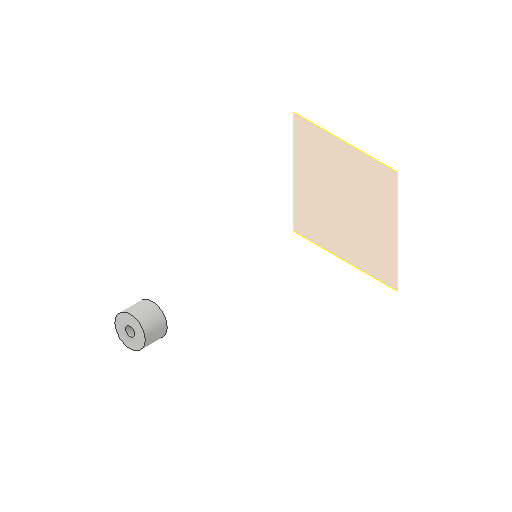
# Autodesk Inventor part: 00_Spacer_13mm
Saved by Autodesk Inventor 2022 (Build 260153000, 153)
## iProperties
Created: 2021-10-19
Part Number: 00_Spacer_13mm
Material: Generic
Document SubType Name: Modeling
Designer: diederichbenedict
Density: 1 g/cm^3
Appearance: Default
Author: diederichbenedict
Autodesk Inventor part; units mm, degrees
ref_plane "YZ Plane" through (0, 0, 0) normal (1, 0, 0) x (0, 1, 0)
ref_plane "XZ Plane" through (0, 0, 0) normal (0, 1, 0) x (-1, 0, 0)
ref_plane "XY Plane" through (0, 0, 0) normal (0, 0, 1) x (1, 0, 0)
ref_plane "Work Plane1" through (458.0192, 138.5867, 202.0511) normal (0, 0, 1) x (1, 0, 0)
sketch "Sketch1" plane through (458.0192, 138.5867, 202.0511) normal (0, 0, 1) x (1, 0, 0)
  circle A0 centre (-101.7255, -104.4963) radius 2.75
  circle A1 centre (-101.7255, -104.4963) radius 9
  point P0 (-458.0192, -138.5867)
  dimension "d0" = 5.5
  dimension "d1" = 18
  constraints: 2 centre point, 1 coincident
  measures "d0" diameter of A0
  measures "d1" diameter of A1
extrude "Extrusion1" add sketch "Sketch1" along normal blind 13
body "Solid1"
